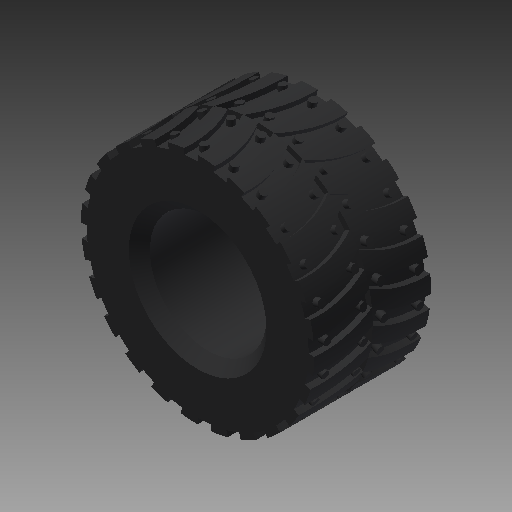
# Autodesk Inventor part: gomallanta
Saved by Autodesk Inventor 2017 (Build 210142000, 142)
## iProperties
Created: 2016-09-08
Part Number: gomallanta
Material: Generic
Document SubType Name: Modeling
Designer: USERPC
Density: 1 g/cm^3
Appearance: Rubber - Black
Author: USERPC
Autodesk Inventor part; units mm, degrees
note: some values were not read from the file. Chosen so that the rebuilt part matches the saved one: direction of "Emboss1".
ref_plane "YZ Plane" through (0, 0, 0) normal (1, 0, 0) x (0, 1, 0)
ref_plane "XY Plane" through (0, 0, 0) normal (0, 0, 1) x (1, 0, 0)
sketch "Sketch1" plane through (0, 0, 0) normal (0, 0, 1) x (1, 0, 0)
  circle A0 centre (0, 0) radius 61
  dimension "d2" = 122
  constraints: 1 centre point
  measures "d2" diameter of A0
extrude "Extrusion1" add sketch "Sketch1" along normal blind 61
sketch "Sketch2" plane through (0, 0, 61) normal (0, 0, 1) x (1, 0, 0)
  circle A0 centre (0, 0) radius 42.5
  circle A1 centre (0, 0) radius 30.5
  dimension "d5" = 85
  dimension "d6" = 61
  constraints: 2 centre point, 2 coincident
  measures "d5" diameter of A0
  measures "d6" diameter of A1
extrude "Extrusion2" cut sketch "Sketch2" against normal blind 104.925 contours A1
chamfer "Chamfer3" distance 5.5 angle 45 1 edges at (-30.5, 0, 61)
chamfer "Chamfer4" distance 5.5 angle 45 1 edges at (-30.5, 0, 0)
ref_plane "Work Plane1" through (0, -61, 0) normal (0, 1, 0) x (-1, 0, 0)
sketch "Sketch3" plane through (0, -61, 0) normal (0, 1, 0) x (-1, 0, 0)
  line L0 (0, 61) -> (-7, 61)
  line L1 (36, 61) -> (-36, 61) projected
  arc A0 (-7, 30.5) -> (0, 61) centre (-50.8359, 56.614) ccw
  arc A1 (-14.8612, 30.5) -> (-7, 61) centre (-57.9283, 57.8633) ccw
  line L2 (-14.8612, 30.5) -> (-21.8612, 30.5)
  line L3 (0, 0) -> (-7, 0)
  line L4 (-36, 0) -> (36, 0) projected
  line L5 (-7, 0) -> (-14, 0)
  line L6 (0, 0) -> (-7, 0)
  arc A2 (-14, 0) -> (-21.8612, 30.5) centre (-71.0131, 1.5683) ccw
  line L7 (61, 61) -> (-61, 61) projected
  line L8 (-61, 0) -> (61, 0) projected
  line L9 (61, 61) -> (-61, 61) projected
  line L10 (-61, 0) -> (61, 0) projected
  arc A3 (-7, 0) -> (-14.8612, 30.5) centre (-64.0131, 1.5683) ccw
  line L11 (-14.8612, 30.5) -> (-7, 30.5)
  arc A4 (-14.8612, 30.5) -> (-7, 61) centre (-57.9283, 57.8633) ccw
  line L12 (30.5, 5.5) -> (-30.5, 5.5) projected
  circle A5 centre (-10.9306, 5.5) radius 2
  circle A6 centre (-14.8612, 24.1638) radius 2
  circle A7 centre (-8.9306, 34.6226) radius 2
  circle A8 centre (-3.5, 53.8997) radius 2
  dimension "d24" = 7
  dimension "d39" = 4
  dimension "d40" = 4
  dimension "d41" = 4
  dimension "d42" = 4
  constraints: 12 end point, 10 point on circle, 9 centre point, 4 point on line, 3 equal radius, 2 horizontal
  measures "d24" distance of L3.start L3.end
  measures "d39" diameter of A5
  measures "d40" diameter of A6
  measures "d41" diameter of A7
  measures "d42" diameter of A8
emboss "Emboss1" sketch "Sketch3" operation cut depth 3 direction (0, 1, 0) contours A0 L11 A1 L0 | A3 L12 A5 A2 L2 | A3 L4 A2 L12 A5
pattern_circular "Circular Pattern1" count 24 over 360 about axis through (0, 0, 0) along (0, 0, 1) of "Emboss1"
body "Solid1"
